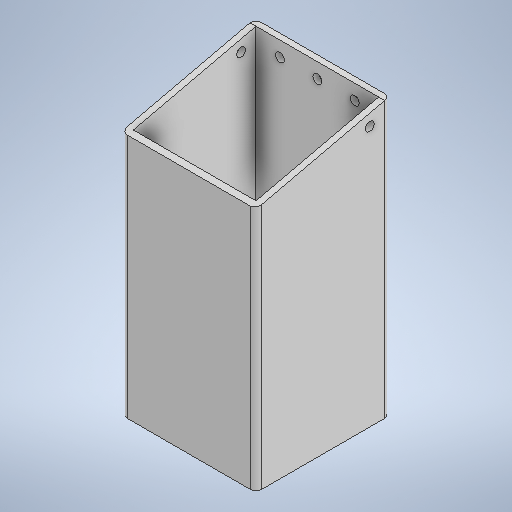
# Autodesk Inventor part: reduced_turtle
Saved by Autodesk Inventor 2025.1 (Build 291241000, 241)
## iProperties
Created: 2025-04-09
Part Number: reduced_turtle
Material: Generic
Document SubType Name: Modeling
Designer: Ian Ching
Density: 1 g/cm^3
Appearance: Default
Author: Ian Ching
Autodesk Inventor part; units mm, degrees
ref_plane "YZ Plane" through (0, 0, 0) normal (1, 0, 0) x (0, 1, 0)
ref_plane "XZ Plane" through (0, 0, 0) normal (0, 1, 0) x (-1, 0, 0)
ref_plane "XY Plane" through (0, 0, 0) normal (0, 0, 1) x (1, 0, 0)
sketch "Sketch1" plane through (0, 0, 0) normal (0, 1, 0) x (-1, 0, 0)
  line L0 (0, 0) -> (45, 0)
  line L1 (45, 0) -> (45, -45)
  line L2 (45, -45) -> (0, -45)
  line L3 (0, -45) -> (0, 0)
  dimension "d0" = 45
  dimension "d1" = 45
  constraints: 8 end point, 2 parallel, 1 horizontal, 1 perpendicular
  measures "d0" distance of L1.end L2.end
  measures "d1" distance of L0.end L1.end
extrude "Extrusion1" add sketch "Sketch1" along normal blind 2
sketch "Sketch2" plane through (0, 2, 0) normal (0, 1, 0) x (1, 0, 0)
  line L0 (-45, 0) -> (0, 0) projected
  line L1 (-22.5, 0) -> (-22.5, 45)
  line L2 (0, 45) -> (-45, 45) projected
  line L3 (0, 0) -> (0, 45) projected
  line L4 (0, 22.5) -> (-45, 22.5)
  line L5 (-45, 45) -> (-45, 0) projected
  line L6 (-43, 2) -> (-2, 2)
  line L7 (-2, 2) -> (-2, 43)
  line L8 (-2, 43) -> (-43, 43)
  line L9 (-43, 43) -> (-43, 2)
  point P0 (-43, 22.5)
  point P1 (-22.5, 43)
  dimension "d10" = 3
  dimension "d4" = 41
  dimension "d5" = 41
  constraints: 12 end point, 6 midpoint, 2 parallel, 2 point on line, 1 horizontal, 1 perpendicular
  measures "d4" distance of L8.end L7.end
  measures "d5" distance of L7.end L6.end
extrude "Extrusion2" add sketch "Sketch2" along normal blind 90 contours L5 L4 L9 L6 L1 L0 | L1 L6 L7 L4 L3 L0 | L5 L2 L1 L8 L9 L4 | L4 L7 L8 L1 L2 L3
sketch "Sketch3" plane through (0, 0, -45) normal (0, 0, -1) x (-1, 0, 0)
  line L0 (45, 0) -> (45, 92) projected
  line L1 (45, 0) -> (20, 0)
  line L2 (20, 0) -> (20, 5)
  line L3 (20, 5) -> (45, 5)
  line L4 (45, 5) -> (45, 0)
  circle A0 centre (20, 5) radius 1.5
  point P0 (0, 0)
  dimension "d8" = 25
  dimension "d9" = 5
  dimension "d10" = 3
  constraints: 8 end point, 2 parallel, 1 centre point, 1 coincident, 1 horizontal, 1 perpendicular
  measures "d8" distance of L2.end L3.end
  measures "d9" distance of L1.end L2.end
  measures "d10" diameter of A0
extrude "Extrusion3" cut sketch "Sketch3" against normal blind 5 contours A0 L2 L3 | L3 L2 A0
fillet "Fillet1" radius 2 4 edges at (0, 46, -45) (-45, 46, -45) (-45, 46, 0) (0, 46, 0)
sketch "Sketch5" plane through (-43, 2, -43) normal (0, 0, 1) x (1, 0, 0)
  line L0 (0, 90) -> (41, 90) projected
  line L1 (-2, 80) -> (20.5, 80)
  line L2 (20.5, 80) -> (20.5, 85)
  line L3 (20.5, 85) -> (-2, 85)
  line L4 (-2, 85) -> (-2, 80)
  line L5 (-2, 80) -> (8, 80)
  line L6 (8, 80) -> (8, 85)
  line L7 (8, 85) -> (-2, 85)
  line L8 (-2, 85) -> (-2, 80)
  line L9 (0, 90) -> (41, 90) projected
  line L10 (43, 80) -> (33, 80)
  line L11 (33, 80) -> (33, 85)
  line L12 (33, 85) -> (43, 85)
  line L13 (43, 85) -> (43, 80)
  circle A0 centre (8, 85) radius 1.5
  circle A1 centre (20.5, 85) radius 1.5
  circle A2 centre (33, 85) radius 1.5
  point P0 (43, -2)
  dimension "d19" = 22.5
  dimension "d20" = 5
  dimension "d21" = 10
  dimension "d22" = 5
  dimension "d23" = 10
  dimension "d24" = 5
  dimension "d25" = 3
  dimension "d26" = 3
  dimension "d27" = 3
  constraints: 24 end point, 6 parallel, 3 centre point, 3 coincident, 3 horizontal, 3 perpendicular, 2 other
  measures "d19" distance of L3.end L2.end
  measures "d20" distance of L2.end L1.end
  measures "d21" distance of L7.end L6.end
  measures "d22" distance of L6.end L5.end
  measures "d23" distance of L11.end L12.end
  measures "d24" distance of L10.end L11.end
  measures "d25" diameter of A0
  measures "d26" diameter of A1
  measures "d27" diameter of A2
extrude "Extrusion5" cut sketch "Sketch5" against normal blind 10 contours A0 L3 L6 | L6 L3 A0 | A0 L3 | A1 L3 L2 | L2 L3 A1 | A2 L12 L11 | L11 L12 A2
sketch "Sketch6" plane through (0, 0, -2) normal (1, 0, 0) x (0, 0, -1)
  line L0 (41, 92) -> (41, 0) projected
  line L1 (-2, 0) -> (-2, 92) projected
  line L2 (41, 92) -> (-2, 92)
  line L3 (-2, 92) -> (-2, 82)
  line L4 (-2, 82) -> (41, 92)
  dimension "d30" = 10
  constraints: 6 end point, 2 perpendicular
  measures "d30" distance of L1.end L3.end
extrude "Extrusion6" cut sketch "Sketch6" against normal blind 90
sketch "Sketch7" plane through (-45, 0, -43) normal (-1, 0, 0) x (0, 0, 1)
  line L0 (0, 2) -> (0, 92) projected
  line L1 (0, 92) -> (5, 92)
  line L2 (5, 92) -> (5, 87)
  line L3 (5, 87) -> (0, 87)
  line L4 (0, 87) -> (0, 92)
  circle A0 centre (5, 87) radius 1.5
  point P0 (43, 0)
  dimension "d33" = 5
  dimension "d34" = 5
  dimension "d35" = 3
  constraints: 8 end point, 2 parallel, 1 centre point, 1 coincident, 1 horizontal, 1 perpendicular
  measures "d33" distance of L2.end L3.end
  measures "d34" distance of L1.end L2.end
  measures "d35" diameter of A0
extrude "Extrusion7" cut sketch "Sketch7" against normal blind 90 contours A0 L2 L3 | L3 L2 A0
body "Solid1"
